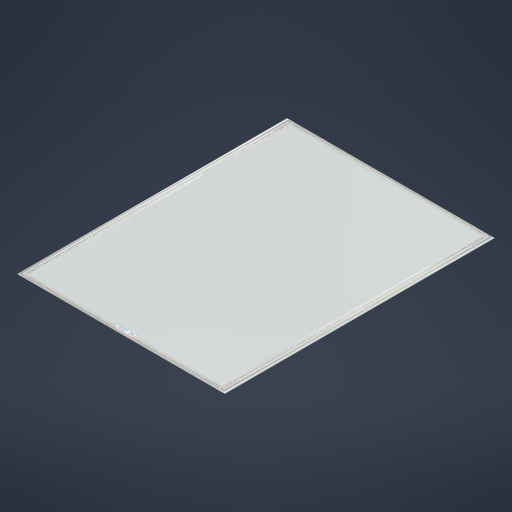
# Autodesk Inventor part: 12inch Touchscreen
Saved by Autodesk Inventor 2023 (Build 270158000, 158)
## iProperties
Created: 2023-02-24
Part Number: 12inch Touchscreen
Material: Glass
Document SubType Name: Modeling
Designer: roota
Density: 2.18 g/cm^3
Appearance: Clear
Author: roota
Autodesk Inventor part; units mm, degrees
ref_plane "YZ Plane" through (0, 0, 0) normal (1, 0, 0) x (0, 1, 0)
ref_plane "XZ Plane" through (0, 0, 0) normal (0, 1, 0) x (-1, 0, 0)
ref_plane "XY Plane" through (0, 0, 0) normal (0, 0, 1) x (1, 0, 0)
sketch "Sketch1" plane through (0, 0, 0) normal (0, 1, 0) x (-1, 0, 0)
  line L0 (100, 130) -> (-100, 130)
  line L1 (-100, 130) -> (-100, -130)
  line L2 (-100, -130) -> (100, -130)
  line L3 (100, -130) -> (100, 130)
  line L4 (100, 130) -> (-100, -130) construction
  line L5 (-100, 130) -> (100, -130) construction
  point P0 (0, 0)
  dimension "d0" = 200
  dimension "d1" = 260
  constraints: 12 end point, 2 midpoint, 2 parallel, 1 horizontal, 1 perpendicular
  measures "d0" distance of L2.end L1.end
  measures "d1" distance of L1.end L0.end
extrude "Extrusion1" add sketch "Sketch1" along normal blind 0.188
sketch "Sketch10" plane through (0, 0.188, 0) normal (0, 1, 0) x (1, 0, 0)
  line L0 (98.0274, 130) -> (98.0274, -130) construction
  line L1 (98.0274, -130) -> (-100, -130) construction
  line L2 (-100, -130) -> (-100, 130) construction
  line L3 (-100, 130) -> (98.0274, 130) construction
  point P0 (0, 0)
  constraints: 2 coincident, 2 other
decal "Decal6"
sketch "Sketch9" plane through (0, 0.188, 0) normal (0, 1, 0) x (1, 0, 0)
  line L0 (-9.9844, -128.5553) -> (-9.9844, -122.1467) construction
  line L1 (-9.9844, -122.1467) -> (9.7409, -122.1467) construction
  line L2 (9.7409, -122.1467) -> (9.7409, -128.5553) construction
  line L3 (9.7409, -128.5553) -> (-9.9844, -128.5553) construction
  point P0 (0, 0)
  dimension "d4" = 86.7
  dimension "d10" = 15
  constraints: 2 other
decal "Decal5"
sketch "Sketch3" plane through (0, 0, 0) normal (1, 0, 0) x (0, 1, 0)
  spline S0 degree 4 poles (0, 130) (0, 134.3549) (-9.0593, 147.1572) (-19.4619, 125.9965) (-6.9491, 96.3655) (-6.9491, 83.2036) knots 0 0 0 0 0 0.420826 1 1 1 1 1 projected
  line L0 (0, 130) -> (0, -130) projected
  line L1 (0, 130) -> (0.1, 130)
  line L2 (0, 130) -> (0.188, 130) projected
  line L3 (-6.9491, 83.2036) -> (-7.0491, 83.2036)
  spline S1 degree 5 poles (0.1, 130) (0.0999, 130.7954) (-0.017, 131.5897) (-0.2179, 132.364) (-0.7519, 133.8263) (-1.5559, 135.1598) (-2.0073, 135.7686) (-2.965, 136.7984) (-4.1568, 137.5316) (-4.7548, 137.7872) (-6.0482, 138.0402) (-7.3305, 137.7183) (-7.9237, 137.4056) (-9.164, 136.4631) (-10.0685, 135.179) (-10.4989, 134.3928) (-11.3564, 132.4589) (-11.8922, 130.4106) (-12.1251, 129.2156) (-12.5034, 126.5087) (-12.6139, 123.7764) (-12.6115, 122.2599) (-12.4934, 118.9927) (-12.1716, 115.739) (-11.9539, 113.9995) (-11.4262, 110.3949) (-10.7782, 106.8098) (-10.42, 104.954) (-9.6764, 101.242) (-8.9232, 97.532) (-8.5546, 95.6725) (-7.8843, 92.081) (-7.367, 88.4642) (-7.1705, 86.7173) (-7.0491, 84.9607) (-7.0491, 83.2036) knots 0 0 0 0 0 0 0.057801 0.057801 0.057801 0.112642 0.112642 0.112642 0.158856 0.158856 0.158856 0.206231 0.206231 0.206231 0.271221 0.271221 0.271221 0.359552 0.359552 0.359552 0.469703 0.469703 0.469703 0.597094 0.597094 0.597094 0.734483 0.734483 0.734483 0.872281 0.872281 0.872281 1 1 1 1 1 1
  point P0 (0, 0)
  dimension "d5" = 0.1
  constraints: 8 end point, 2 parallel, 1 horizontal, 1 perpendicular
sketch "Sketch11" plane through (0, 0, 0) normal (0, -1, 0) x (1, 0, 0)
  line L0 (-98.7516, -130.9508) -> (-100, 130) construction
  line L1 (-100, 130) -> (98.7516, 130.9508) construction
  line L2 (98.7516, 130.9508) -> (100, -130) construction
  line L3 (100, -130) -> (-98.7516, -130.9508) construction
  point P0 (0, 0)
  constraints: 2 coincident, 2 other
sketch "Sketch5" plane through (0, 0.188, 0) normal (0, 1, 0) x (1, 0, 0)
  line L0 (7.5, -44.1487) -> (7.5, -140.6515) construction
  line L1 (7.5, -140.6515) -> (-7.5, -140.6515) construction
  line L2 (-7.5, -140.6515) -> (-7.5, -44.1487) construction
  line L3 (-7.5, -44.1487) -> (7.5, -44.1487) construction
  point P0 (0, 0)
  point P1 (7.5, -130)
  point P2 (-7.5, -130)
  constraints: 2 vertical alignment, 2 other
sketch "Sketch6" plane through (-7.5, -7.0491, 83.2036) normal (0, -1, 0) x (1, 0, 0)
  line L0 (0.0146, -20.011) -> (0, 0) construction
  line L1 (0, 0) -> (14.9854, 0.011) construction
  line L2 (14.9854, 0.011) -> (15, -20) construction
  line L3 (15, -20) -> (0.0146, -20.011) construction
  point P0 (7.5, -83.2036)
  point P1 (15, -20)
  constraints: 2 coincident, 2 other
sketch "Sketch7" plane through (7.5, -6.9491, 83.2036) normal (0, 1, 0) x (-1, 0, 0)
  line L0 (0.0146, -20.011) -> (0, 0) construction
  line L1 (0, 0) -> (14.9854, 0.011) construction
  line L2 (14.9854, 0.011) -> (15, -20) construction
  line L3 (15, -20) -> (0.0146, -20.011) construction
  point P0 (7.5, -83.2036)
  point P1 (15, -20)
  constraints: 2 coincident, 2 other
sketch "Sketch8" plane through (0, 0, 0) normal (0, -1, 0) x (1, 0, 0)
  line L0 (7.5, 207.6879) -> (7.5, 130) construction
  line L1 (7.5, 130) -> (-7.5, 130) construction
  line L2 (-7.5, 130) -> (-7.5, 207.6879) construction
  line L3 (-7.5, 207.6879) -> (7.5, 207.6879) construction
  point P0 (0, 0)
  constraints: 4 end point
sketch "Sketch13" plane through (0, -36.5283, 83.3447) normal (0, -0.9338373, 0.3576979) x (1, 0, 0)
  line L0 (7.5, 88.1007) -> (7.5, 10.4128) construction
  line L1 (7.5, 10.4128) -> (-7.5, 10.4128) construction
  line L2 (-7.5, 10.4128) -> (-7.5, 88.1007) construction
  line L3 (-7.5, 88.1007) -> (7.5, 88.1007) construction
  point P0 (0, -64.7643)
  constraints: 2 coincident, 2 other
body "Solid1"
